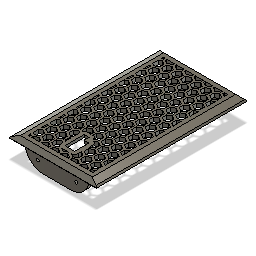
Compact_Robot_MB4 v1 (Autodesk Fusion 360 design; units mm, degrees)
Autodesk Fusion 360 part; units mm, degrees
(part 1 of 2)
sketch "Sketch1" plane through (0, 0, 0) normal (0, 1, 0) x (1, 0, 0)
  line L0 (23.335, 40.235) -> (-23.335, 40.235)
  line L1 (-23.335, 40.235) -> (-23.335, -40.235)
  line L2 (-23.335, -40.235) -> (23.335, -40.235)
  line L3 (23.335, -40.235) -> (23.335, 40.235)
  line L4 (23.335, 40.235) -> (-23.335, -40.235) construction
  line L5 (-23.335, 40.235) -> (23.335, -40.235) construction
  dimension "d1" = 80.47
  dimension "d2" = 46.67
  constraint horizontal L0
  constraint perpendicular L0 L1
  constraint parallel L0 L2
  constraint parallel L1 L3
  constraint coincident L4 origin
  constraint coincident L5 origin
  measures "d1" distance of L0.end L1.end
  measures "d2" distance of L1.end L2.end
extrude "Extrude1" add sketch "Sketch1" along normal blind 2.12
sketch "Sketch2" plane through (0, 0, 0) normal (0, 0, 1) x (1, 0, 0)
  line L0 (-27, 0) -> (28.2654, 0)
  circle A0 centre (-7.215, 0) radius 10
  circle A1 centre (7.215, 0) radius 10
  line L1 (-7.215, -10) -> (7.215, -10)
  line L2 (23.335, 0) -> (23.335, 2.12)
  circle A2 centre (10.2519, -5) radius 0.75
  circle A3 centre (-10.2581, -5) radius 0.75
  dimension "d5" = 20
  dimension "d6" = 20
  dimension "d7" = 14.43
  dimension "d8" = 16.12
  dimension "d12" = 1.5
  dimension "d13" = 1.5
  dimension "d14" = 10
  dimension "d15" = 10
  dimension "d16" = 20.51
  dimension "d17" = 5.85
  constraint horizontal L0
  constraint coincident L0 A0.centre
  constraint coincident L0 A1.centre
  constraint horizontal origin A0.centre
  constraint coincident A1 L1.end
  constraint tangent A1 L1
  constraint tangent A0 L1
  constraint coincident A0 L1.start
  measures "d5" diameter of A0
  measures "d6" diameter of A1
  measures "d7" distance of L1.start L1.end
  measures "d8" distance of A1.centre L2
  measures "d12" diameter of A2
  measures "d13" diameter of A3
  measures "d16" distance of A2.centre A3.centre
  measures "d17" distance of A1.centre A2.centre
extrude "Extrude2" add sketch "Sketch2" along normal blind 1.8 from surface at 36.03 contours L0 A0 A1 | L0 A0 A1 | L0 A0 A1 | A0 A1 L1 picked at (-0.9013, -0.4238) picked at (10.0653, -1.4174) picked at (-10.0674, -1.4174)
extrude "Extrude3" add sketch "Sketch2" along normal blind 1.8 from surface at -37.83 contours L0 A0 A1 | L0 A0 A1 | L0 A0 A1 | A0 A1 L1 picked at (-0.9013, -0.4238) picked at (10.0653, -1.4174) picked at (-10.0674, -1.4174)
sketch "Sketch3" plane through (0, 0, 0) normal (0, 0, 1) x (1, 0, 0)
  line L0 (19.209, 2.12) -> (22.6292, 0.7084)
  line L1 (22.6292, 0.7084) -> (23.335, 0)
  line L2 (-23.335, 2.12) -> (23.335, 2.12)
  line L3 (19.209, 2.12) -> (20.385, 0.1201)
  line L4 (20.385, 0.1201) -> (22.6292, 0.7084)
  line L5 (20.385, 0.1201) -> (20.5053, 0)
  line L6 (-23.335, 0) -> (23.335, 0)
  line L7 (-19.209, 2.12) -> (-22.6292, 0.7084)
  line L8 (-22.6292, 0.7084) -> (-23.335, 0)
  line L9 (-22.6292, 0.7084) -> (-20.385, 0.1201)
  line L10 (-20.385, 0.1201) -> (-19.209, 2.12)
  line L11 (-20.385, 0.1201) -> (-20.5053, 0)
  line L12 (-20.385, 0.1201) -> (20.385, 0.1201)
  line L13 (-23.335, 2.12) -> (-23.335, 0)
  line L14 (-23.335, 2.12) -> (23.335, 2.12)
  line L15 (23.335, 2.12) -> (23.335, 0)
  point P0 (23.335, 0)
  dimension "d21" = 3.7
  dimension "d22" = 1
  dimension "d23" = 2.32
  dimension "d24" = 2.32
  dimension "d25" = 0.17
  dimension "d26" = 3.7
  dimension "d27" = 1
  dimension "d28" = 2.32
  dimension "d29" = 2.32
  dimension "d30" = 0.17
  dimension "d31" = 40.77
  constraint coincident P0 L1.end
  constraint coincident L0.start L2
  constraint coincident L5.end L6
  constraint coincident L2 L7.start
  constraint coincident L6.start L8.end
  constraint coincident L6 L11.end
  constraint horizontal L12
  constraint coincident L2.start L13.start
  constraint coincident L2.end L14.end
  measures "d21" distance of L0.start L0.end
  measures "d22" distance of L0.end P0
  measures "d23" distance of L0.start L3.end
  measures "d24" distance of L0.end L3.end
  measures "d25" distance of L3.end L5.end
  measures "d26" distance of L7.start L7.end
  measures "d27" distance of L7.end L6.start
  measures "d28" distance of L7.end L9.end
  measures "d29" distance of L7.start L9.end
  measures "d30" distance of L9.end L11.end
  measures "d31" horizontal distance of L3.end L9.end
extrude "Extrude4" cut sketch "Sketch3" along normal through all and the other way through all contours L0 L1 L2 L14 L15 | L2 L7 L8 L13 L14
sketch "Sketch4" plane through (0, 0, 0) normal (1, 0, 0) x (0, 0, -1)
  line L0 (-40.235, 0.12) -> (-38.2328, 0.7084)
  line L1 (-40.235, 0.12) -> (-38.2328, 2.12)
  line L2 (-38.2328, 2.12) -> (-38.2328, 0.7084)
  line L3 (40.235, 0.7084) -> (-40.235, 0.7084)
  line L4 (-40.235, 2.12) -> (40.235, 2.12)
  line L5 (-40.235, 0) -> (-40.235, 0.7084)
  line L6 (0, 0) -> (0, 5)
  line L7 (38.2328, 2.12) -> (38.2328, 0.7084)
  line L8 (40.235, 0.12) -> (38.2328, 2.12)
  line L9 (40.235, 0.12) -> (38.2328, 0.7084)
  line L10 (-40.235, 0.12) -> (-40.235, 2.12)
  line L11 (-38.2328, 2.12) -> (-40.235, 2.12)
  line L12 (40.235, 0.12) -> (40.235, 2.12)
  line L13 (38.2328, 2.12) -> (40.235, 2.12)
  dimension "d34" = 2.83
  dimension "d36" = 0.12
  constraint vertical L2
  constraint coincident L0.end L3
  constraint coincident L1.end L4
  constraint coincident L0.start L5
  constraint coincident L0.start L1.start
  constraint coincident L6.start origin
  constraint perpendicular L4 L6
  constraint symmetric L0.start L6 L8.start
  constraint symmetric L0.end L6 L7.end
  constraint symmetric L1.end L6 L7.start
  constraint coincident L4.start L10.end
  constraint coincident L4.end L12.end
  measures "d34" distance of L0.start L1.end
  measures "d36" distance of L0.start L5.start
extrude "Extrude5" cut sketch "Sketch4" along normal through all and the other way through all contours L1 L3 L5 L10 | L1 L3 L4 L10 L11 | L3 L4 L8 L12 L13 | L3 L8 L12
sketch "Sketch5" plane through (0, 2.12, 0) normal (0, 1, 0) x (-1, 0, 0)
  line L0 (-19.209, -38.2328) -> (19.209, -38.2328)
  line L1 (19.209, -38.2328) -> (19.209, 38.2328)
  line L2 (19.209, 38.2328) -> (-19.209, 38.2328)
  line L3 (-19.209, 38.2328) -> (-19.209, -38.2328)
  line L4 (-17.21, -36.03) -> (17.21, -36.03)
  line L5 (17.21, -36.03) -> (17.21, 36.03)
  line L6 (17.21, 36.03) -> (-17.21, 36.03)
  line L7 (-17.21, 36.03) -> (-17.21, -36.03)
  line L8 (-17.21, -36.03) -> (17.21, 36.03) construction
  line L9 (17.21, -36.03) -> (-17.21, 36.03) construction
  line L10 (-0.69, -20.08) -> (3.31, -20.08)
  line L11 (3.31, -20.08) -> (3.31, -31.73)
  line L12 (3.31, -31.73) -> (-3.29, -31.73)
  line L13 (-3.29, -31.73) -> (-3.29, -22.73)
  line L14 (2.61, -20.78) -> (0.01, -20.78)
  line L15 (0.01, -20.78) -> (0.01, -23.43)
  line L16 (2.61, -31.03) -> (2.61, -20.78)
  line L17 (2.61, -31.03) -> (-2.59, -31.03)
  line L18 (-2.59, -31.03) -> (-2.59, -23.43)
  line L19 (-2.59, -23.43) -> (0.01, -23.43)
  line L20 (-3.29, -22.73) -> (-0.69, -22.73)
  line L21 (-0.69, -22.73) -> (-0.69, -20.08)
  line L22 (25, 0) -> (0, 0)
  line L23 (2.61, 31.03) -> (2.61, 20.78)
  line L24 (-2.59, 31.03) -> (-2.59, 23.43)
  line L25 (-0.69, 22.73) -> (-0.69, 20.08)
  line L26 (0.01, 20.78) -> (0.01, 23.43)
  line L27 (3.31, 20.08) -> (3.31, 31.73)
  line L28 (2.61, 20.78) -> (0.01, 20.78)
  line L29 (-3.29, 31.73) -> (-3.29, 22.73)
  line L30 (-2.59, 23.43) -> (0.01, 23.43)
  line L31 (2.61, 31.03) -> (-2.59, 31.03)
  line L32 (-3.29, 22.73) -> (-0.69, 22.73)
  line L33 (3.31, 31.73) -> (-3.29, 31.73)
  line L34 (-0.69, 20.08) -> (3.31, 20.08)
  line L35 (2.61, 33.03) -> (-2.59, 33.03)
  line L36 (-4.59, 31.03) -> (-4.59, 23.43)
  line L37 (-1.99, 21.43) -> (-2.59, 21.43)
  line L38 (-1.99, 21.43) -> (-1.99, 20.78)
  line L39 (4.61, 31.03) -> (4.61, 20.78)
  line L40 (2.61, 18.78) -> (0.01, 18.78)
  arc A0 (4.61, 31.03) -> (2.61, 33.03) centre (2.61, 31.03) ccw
  arc A1 (2.61, 18.78) -> (4.61, 20.78) centre (2.61, 20.78) ccw
  arc A2 (-1.99, 20.78) -> (0.01, 18.78) centre (0.01, 20.78) ccw
  arc A3 (-4.59, 23.43) -> (-2.59, 21.43) centre (-2.59, 23.43) ccw
  arc A4 (-2.59, 33.03) -> (-4.59, 31.03) centre (-2.59, 31.03) ccw
  dimension "d40" = 72.06
  dimension "d41" = 34.42
  dimension "d42" = 0.7
  dimension "d44" = 0.7
  dimension "d46" = 0.7
  dimension "d47" = 0.7
  dimension "d49" = 2.6
  dimension "d51" = 0.7
  dimension "d52" = 7.6
  dimension "d53" = 0.7
  dimension "d54" = 10.25
  dimension "d55" = 5.2
  dimension "d56" = 5
  dimension "d57" = 14.62
  dimension "d63" = 1.3
  dimension "d64" = 1.3
  dimension "d65" = 1.3
  dimension "d66" = 1.3
  dimension "d67" = 1.3
  dimension "d68" = 1.3
  dimension "d69" = 2
  dimension "d70" = 2
  dimension "d71" = 2
  dimension "d72" = 2
  dimension "d73" = 2
  constraint horizontal L4
  constraint perpendicular L4 L5
  constraint parallel L4 L6
  constraint parallel L5 L7
  constraint coincident L8 L22.end
  constraint coincident L9 L22.end
  constraint coincident L22.end origin
  constraint horizontal L10
  constraint vertical L11
  constraint horizontal L12
  constraint vertical L13
  constraint horizontal L20
  constraint horizontal L14
  constraint vertical L15
  constraint vertical L16
  constraint horizontal L17
  constraint vertical L18
  constraint horizontal L19
  constraint perpendicular L3 L22
  constraint symmetric L11.end L22 L27.end
  constraint symmetric L10.start L22 L25.end
  constraint symmetric L10.end L22 L27.start
  constraint symmetric L12.end L22 L29.start
  constraint symmetric L13.end L22 L29.end
  constraint symmetric L14.start L22 L23.end
  constraint symmetric L14.end L22 L26.start
  constraint symmetric L16.start L22 L23.start
  constraint symmetric L17.end L22 L24.start
  constraint symmetric L18.end L22 L24.end
  constraint symmetric L15.end L22 L26.end
  constraint symmetric L20.end L22 L25.start
  constraint horizontal L35
  constraint perpendicular L6 L36
  constraint horizontal L37
  constraint parallel L25 L38
  constraint vertical L39
  constraint perpendicular L39 L40
  constraint tangent L39 A0
  constraint tangent L40 A1
  constraint tangent L38 A2
  constraint tangent L36 A4
  constraint tangent L35 A0
  constraint tangent L35 A4
  constraint tangent L36 A3
  constraint tangent L40 A2
  constraint tangent L37 A3
  constraint tangent L39 A1
  measures "d40" distance of L4.start L6.end
  measures "d41" distance of L5.end L6.end
  measures "d42" distance of L11 L16
  measures "d44" distance of L10 L14
  measures "d46" distance of L19 L20
  measures "d47" distance of L13 L18
  measures "d49" distance of L15 L16
  measures "d51" distance of L15 L21
  measures "d52" distance of L17 L19
  measures "d53" distance of L12 L17
  measures "d54" distance of L14 L17
  measures "d55" distance of L16 L18
  measures "d56" distance of L4 L17
  measures "d57" distance of L7 L18
  measures "d63" distance of L33 L35
  measures "d64" distance of L27 L39
  measures "d65" distance of L29 L36
  measures "d66" distance of L32 L37
  measures "d67" distance of L25 L38
  measures "d68" distance of L34 L40
  measures "d69" radius of A0
  measures "d70" radius of A1
  measures "d71" radius of A2
  measures "d72" radius of A3
  measures "d73" radius of A4
extrude "Extrude6" cut sketch "Sketch5" against normal through all contours L23 L24 L26 L28 L30 L31
extrude "Extrude7" cut sketch "Sketch5" along normal blind 0.7 from surface at -2.12 contours L25 L27 L29 L32 L33 L34
chamfer "Chamfer1" distance 0.7 angle 45 6 edges at (3.29, 0.7, 27.23) (-0.01, 0.7, 31.73) (-3.31, 0.7, 25.905) (1.99, 0.7, 22.73) (0.69, 0.7, 21.405) (-1.31, 0.7, 20.08)
sketch "Sketch6" plane through (0, 2.12, 0) normal (0, 1, 0) x (-1, 0, 0)
  line L0 (0.01, 20.78) -> (0.01, 23.43)
  line L1 (0.01, 23.43) -> (-2.59, 23.43)
  line L2 (-2.59, 23.43) -> (-2.59, 31.03)
  line L3 (-2.59, 31.03) -> (2.61, 31.03)
  line L4 (2.61, 31.03) -> (2.61, 20.78)
  line L5 (2.61, 20.78) -> (0.01, 20.78)
  line L6 (-19.209, -38.2328) -> (19.209, -38.2328)
  line L7 (19.209, -38.2328) -> (19.209, 38.2328)
  line L8 (19.209, 38.2328) -> (-19.209, 38.2328)
  line L9 (-19.209, 38.2328) -> (-19.209, -38.2328)
  line L10 (17.209, 36.0228) -> (17.209, -36.0228)
  line L11 (17.209, -36.0228) -> (-17.209, -36.0228)
  line L12 (-17.209, -36.0228) -> (-17.209, 36.0228)
  line L13 (-17.209, 36.0228) -> (17.209, 36.0228)
  line L14 (16.459, 37.5128) -> (16.459, 35.2028)
  line L15 (16.459, 35.2028) -> (18.4596, 34.0478)
  line L16 (18.4596, 34.0478) -> (20.4601, 35.2028)
  line L17 (20.4601, 35.2028) -> (20.4601, 37.5128)
  line L18 (20.4601, 37.5128) -> (18.4596, 38.6678)
  line L19 (18.4596, 38.6678) -> (16.459, 37.5128)
  line L20 (16.459, 28.4168) -> (16.459, 26.1068)
  line L21 (16.459, 26.1068) -> (18.4596, 24.9518)
  line L22 (18.4596, 24.9518) -> (20.4601, 26.1068)
  line L23 (20.4601, 26.1068) -> (20.4601, 28.4168)
  line L24 (20.4601, 28.4168) -> (18.4596, 29.5718)
  line L25 (18.4596, 29.5718) -> (16.459, 28.4168)
  line L26 (18.4596, 20.4758) -> (16.459, 19.3208)
  line L27 (16.459, 19.3208) -> (16.459, 17.0108)
  line L28 (16.459, 17.0108) -> (18.4596, 15.8558)
  line L29 (18.4596, 15.8558) -> (20.4601, 17.0108)
  line L30 (20.4601, 17.0108) -> (20.4601, 19.3208)
  line L31 (20.4601, 19.3208) -> (18.4596, 20.4758)
  line L32 (18.4596, 11.3798) -> (16.459, 10.2248)
  line L33 (16.459, 10.2248) -> (16.459, 7.9148)
  line L34 (16.459, 7.9148) -> (18.4596, 6.7598)
  line L35 (18.4596, 6.7598) -> (20.4601, 7.9148)
  line L36 (20.4601, 7.9148) -> (20.4601, 10.2248)
  line L37 (20.4601, 10.2248) -> (18.4596, 11.3798)
  line L38 (18.4596, 2.2838) -> (16.459, 1.1288)
  line L39 (16.459, 1.1288) -> (16.459, -1.1812)
  line L40 (16.459, -1.1812) -> (18.4596, -2.3362)
  line L41 (18.4596, -2.3362) -> (20.4601, -1.1812)
  line L42 (20.4601, -1.1812) -> (20.4601, 1.1288)
  line L43 (20.4601, 1.1288) -> (18.4596, 2.2838)
  line L44 (18.4596, -6.8122) -> (16.459, -7.9672)
  line L45 (16.459, -7.9672) -> (16.459, -10.2772)
  line L46 (16.459, -10.2772) -> (18.4596, -11.4322)
  line L47 (18.4596, -11.4322) -> (20.4601, -10.2772)
  line L48 (20.4601, -10.2772) -> (20.4601, -7.9672)
  line L49 (20.4601, -7.9672) -> (18.4596, -6.8122)
  line L50 (18.4596, -15.9082) -> (16.459, -17.0632)
  line L51 (16.459, -17.0632) -> (16.459, -19.3732)
  line L52 (16.459, -19.3732) -> (18.4596, -20.5282)
  line L53 (18.4596, -20.5282) -> (20.4601, -19.3732)
  line L54 (20.4601, -19.3732) -> (20.4601, -17.0632)
  line L55 (20.4601, -17.0632) -> (18.4596, -15.9082)
  line L56 (18.4596, -25.0042) -> (16.459, -26.1592)
  line L57 (16.459, -26.1592) -> (16.459, -28.4692)
  line L58 (16.459, -28.4692) -> (18.4596, -29.6242)
  line L59 (18.4596, -29.6242) -> (20.4601, -28.4692)
  line L60 (20.4601, -28.4692) -> (20.4601, -26.1592)
  line L61 (20.4601, -26.1592) -> (18.4596, -25.0042)
  line L62 (18.4596, -34.1002) -> (16.459, -35.2552)
  line L63 (16.459, -35.2552) -> (16.459, -37.5652)
  line L64 (16.459, -37.5652) -> (18.4596, -38.7202)
  line L65 (18.4596, -38.7202) -> (20.4601, -37.5652)
  line L66 (20.4601, -37.5652) -> (20.4601, -35.2552)
  line L67 (20.4601, -35.2552) -> (18.4596, -34.1002)
  line L68 (13.3396, 29.5718) -> (11.339, 28.4168)
  line L69 (11.339, 28.4168) -> (11.339, 26.1068)
  line L70 (11.339, 26.1068) -> (13.3396, 24.9518)
  line L71 (13.3396, 24.9518) -> (15.3401, 26.1068)
  line L72 (15.3401, 26.1068) -> (15.3401, 28.4168)
  line L73 (15.3401, 28.4168) -> (13.3396, 29.5718)
  line L74 (13.3396, 38.6678) -> (11.339, 37.5128)
  line L75 (11.339, 37.5128) -> (11.339, 35.2028)
  line L76 (11.339, 35.2028) -> (13.3396, 34.0478)
  line L77 (13.3396, 34.0478) -> (15.3401, 35.2028)
  line L78 (15.3401, 35.2028) -> (15.3401, 37.5128)
  line L79 (15.3401, 37.5128) -> (13.3396, 38.6678)
  line L80 (8.2196, 29.5718) -> (6.219, 28.4168)
  line L81 (6.219, 28.4168) -> (6.219, 26.1068)
  line L82 (6.219, 26.1068) -> (8.2196, 24.9518)
  line L83 (8.2196, 24.9518) -> (10.2201, 26.1068)
  line L84 (10.2201, 26.1068) -> (10.2201, 28.4168)
  line L85 (10.2201, 28.4168) -> (8.2196, 29.5718)
  line L86 (8.2196, 38.6678) -> (6.219, 37.5128)
  line L87 (6.219, 37.5128) -> (6.219, 35.2028)
  line L88 (6.219, 35.2028) -> (8.2196, 34.0478)
  line L89 (8.2196, 34.0478) -> (10.2201, 35.2028)
  line L90 (10.2201, 35.2028) -> (10.2201, 37.5128)
  line L91 (10.2201, 37.5128) -> (8.2196, 38.6678)
  line L92 (3.0996, 29.5718) -> (1.099, 28.4168)
  line L93 (1.099, 28.4168) -> (1.099, 26.1068)
  line L94 (1.099, 26.1068) -> (3.0996, 24.9518)
  line L95 (3.0996, 24.9518) -> (5.1001, 26.1068)
  line L96 (5.1001, 26.1068) -> (5.1001, 28.4168)
  line L97 (5.1001, 28.4168) -> (3.0996, 29.5718)
  line L98 (3.0996, 38.6678) -> (1.099, 37.5128)
  line L99 (1.099, 37.5128) -> (1.099, 35.2028)
  line L100 (1.099, 35.2028) -> (3.0996, 34.0478)
  line L101 (3.0996, 34.0478) -> (5.1001, 35.2028)
  line L102 (5.1001, 35.2028) -> (5.1001, 37.5128)
  line L103 (5.1001, 37.5128) -> (3.0996, 38.6678)
  line L104 (-2.0204, 29.5718) -> (-4.021, 28.4168)
  line L105 (-4.021, 28.4168) -> (-4.021, 26.1068)
  line L106 (-4.021, 26.1068) -> (-2.0204, 24.9518)
  line L107 (-2.0204, 24.9518) -> (-0.0199, 26.1068)
  line L108 (-0.0199, 26.1068) -> (-0.0199, 28.4168)
  line L109 (-0.0199, 28.4168) -> (-2.0204, 29.5718)
  line L110 (-2.0204, 38.6678) -> (-4.021, 37.5128)
  line L111 (-4.021, 37.5128) -> (-4.021, 35.2028)
  line L112 (-4.021, 35.2028) -> (-2.0204, 34.0478)
  line L113 (-2.0204, 34.0478) -> (-0.0199, 35.2028)
  line L114 (-0.0199, 35.2028) -> (-0.0199, 37.5128)
  line L115 (-0.0199, 37.5128) -> (-2.0204, 38.6678)
  line L116 (-7.1404, 29.5718) -> (-9.141, 28.4168)
  line L117 (-9.141, 28.4168) -> (-9.141, 26.1068)
  line L118 (-9.141, 26.1068) -> (-7.1404, 24.9518)
  line L119 (-7.1404, 24.9518) -> (-5.1399, 26.1068)
  line L120 (-5.1399, 26.1068) -> (-5.1399, 28.4168)
  line L121 (-5.1399, 28.4168) -> (-7.1404, 29.5718)
  line L122 (-7.1404, 38.6678) -> (-9.141, 37.5128)
  line L123 (-9.141, 37.5128) -> (-9.141, 35.2028)
  line L124 (-9.141, 35.2028) -> (-7.1404, 34.0478)
  line L125 (-7.1404, 34.0478) -> (-5.1399, 35.2028)
  line L126 (-5.1399, 35.2028) -> (-5.1399, 37.5128)
  line L127 (-5.1399, 37.5128) -> (-7.1404, 38.6678)
  line L128 (-12.2604, 29.5718) -> (-14.261, 28.4168)
  line L129 (-14.261, 28.4168) -> (-14.261, 26.1068)
  line L130 (-14.261, 26.1068) -> (-12.2604, 24.9518)
  line L131 (-12.2604, 24.9518) -> (-10.2599, 26.1068)
  line L132 (-10.2599, 26.1068) -> (-10.2599, 28.4168)
  line L133 (-10.2599, 28.4168) -> (-12.2604, 29.5718)
  line L134 (-12.2604, 38.6678) -> (-14.261, 37.5128)
  line L135 (-14.261, 37.5128) -> (-14.261, 35.2028)
  line L136 (-14.261, 35.2028) -> (-12.2604, 34.0478)
  line L137 (-12.2604, 34.0478) -> (-10.2599, 35.2028)
  line L138 (-10.2599, 35.2028) -> (-10.2599, 37.5128)
  line L139 (-10.2599, 37.5128) -> (-12.2604, 38.6678)
  line L140 (-17.3804, 29.5718) -> (-19.381, 28.4168)
  line L141 (-19.381, 28.4168) -> (-19.381, 26.1068)
  line L142 (-19.381, 26.1068) -> (-17.3804, 24.9518)
  line L143 (-17.3804, 24.9518) -> (-15.3799, 26.1068)
  line L144 (-15.3799, 26.1068) -> (-15.3799, 28.4168)
  line L145 (-15.3799, 28.4168) -> (-17.3804, 29.5718)
  line L146 (-17.3804, 38.6678) -> (-19.381, 37.5128)
  line L147 (-19.381, 37.5128) -> (-19.381, 35.2028)
  line L148 (-19.381, 35.2028) -> (-17.3804, 34.0478)
  line L149 (-17.3804, 34.0478) -> (-15.3799, 35.2028)
  line L150 (-15.3799, 35.2028) -> (-15.3799, 37.5128)
  line L151 (-15.3799, 37.5128) -> (-17.3804, 38.6678)
  line L152 (18.4596, 29.5718) -> (16.459, 28.4168)
  line L153 (16.459, 28.4168) -> (16.459, 26.1068)
  line L154 (16.459, 26.1068) -> (18.4596, 24.9518)
  line L155 (18.4596, 24.9518) -> (20.4601, 26.1068)
  line L156 (20.4601, 26.1068) -> (20.4601, 28.4168)
  line L157 (20.4601, 28.4168) -> (18.4596, 29.5718)
  line L158 (13.3396, 20.4758) -> (11.339, 19.3208)
  line L159 (11.339, 19.3208) -> (11.339, 17.0108)
  line L160 (11.339, 17.0108) -> (13.3396, 15.8558)
  line L161 (13.3396, 15.8558) -> (15.3401, 17.0108)
  line L162 (15.3401, 17.0108) -> (15.3401, 19.3208)
  line L163 (15.3401, 19.3208) -> (13.3396, 20.4758)
  line L164 (13.3396, 29.5718) -> (11.339, 28.4168)
  line L165 (11.339, 28.4168) -> (11.339, 26.1068)
  line L166 (11.339, 26.1068) -> (13.3396, 24.9518)
  line L167 (13.3396, 24.9518) -> (15.3401, 26.1068)
  line L168 (15.3401, 26.1068) -> (15.3401, 28.4168)
  line L169 (15.3401, 28.4168) -> (13.3396, 29.5718)
  line L170 (8.2196, 20.4758) -> (6.219, 19.3208)
  line L171 (6.219, 19.3208) -> (6.219, 17.0108)
  line L172 (6.219, 17.0108) -> (8.2196, 15.8558)
  line L173 (8.2196, 15.8558) -> (10.2201, 17.0108)
  line L174 (10.2201, 17.0108) -> (10.2201, 19.3208)
  line L175 (10.2201, 19.3208) -> (8.2196, 20.4758)
  line L176 (8.2196, 29.5718) -> (6.219, 28.4168)
  line L177 (6.219, 28.4168) -> (6.219, 26.1068)
  line L178 (6.219, 26.1068) -> (8.2196, 24.9518)
  line L179 (8.2196, 24.9518) -> (10.2201, 26.1068)
  line L180 (10.2201, 26.1068) -> (10.2201, 28.4168)
  line L181 (10.2201, 28.4168) -> (8.2196, 29.5718)
  line L182 (3.0996, 20.4758) -> (1.099, 19.3208)
  line L183 (1.099, 19.3208) -> (1.099, 17.0108)
  line L184 (1.099, 17.0108) -> (3.0996, 15.8558)
  line L185 (3.0996, 15.8558) -> (5.1001, 17.0108)
  line L186 (5.1001, 17.0108) -> (5.1001, 19.3208)
  line L187 (5.1001, 19.3208) -> (3.0996, 20.4758)
  line L188 (3.0996, 29.5718) -> (1.099, 28.4168)
  line L189 (1.099, 28.4168) -> (1.099, 26.1068)
  line L190 (1.099, 26.1068) -> (3.0996, 24.9518)
  line L191 (3.0996, 24.9518) -> (5.1001, 26.1068)
  line L192 (5.1001, 26.1068) -> (5.1001, 28.4168)
  line L193 (5.1001, 28.4168) -> (3.0996, 29.5718)
  line L194 (-2.0204, 20.4758) -> (-4.021, 19.3208)
  line L195 (-4.021, 19.3208) -> (-4.021, 17.0108)
  line L196 (-4.021, 17.0108) -> (-2.0204, 15.8558)
  line L197 (-2.0204, 15.8558) -> (-0.0199, 17.0108)
  line L198 (-0.0199, 17.0108) -> (-0.0199, 19.3208)
  line L199 (-0.0199, 19.3208) -> (-2.0204, 20.4758)
  line L200 (-2.0204, 29.5718) -> (-4.021, 28.4168)
  line L201 (-4.021, 28.4168) -> (-4.021, 26.1068)
  line L202 (-4.021, 26.1068) -> (-2.0204, 24.9518)
  line L203 (-2.0204, 24.9518) -> (-0.0199, 26.1068)
  line L204 (-0.0199, 26.1068) -> (-0.0199, 28.4168)
  line L205 (-0.0199, 28.4168) -> (-2.0204, 29.5718)
  line L206 (-7.1404, 20.4758) -> (-9.141, 19.3208)
  line L207 (-9.141, 19.3208) -> (-9.141, 17.0108)
  line L208 (-9.141, 17.0108) -> (-7.1404, 15.8558)
  line L209 (-7.1404, 15.8558) -> (-5.1399, 17.0108)
  line L210 (-5.1399, 17.0108) -> (-5.1399, 19.3208)
  line L211 (-5.1399, 19.3208) -> (-7.1404, 20.4758)
  line L212 (-7.1404, 29.5718) -> (-9.141, 28.4168)
  line L213 (-9.141, 28.4168) -> (-9.141, 26.1068)
  line L214 (-9.141, 26.1068) -> (-7.1404, 24.9518)
  line L215 (-7.1404, 24.9518) -> (-5.1399, 26.1068)
  line L216 (-5.1399, 26.1068) -> (-5.1399, 28.4168)
  line L217 (-5.1399, 28.4168) -> (-7.1404, 29.5718)
  line L218 (-12.2604, 20.4758) -> (-14.261, 19.3208)
  line L219 (-14.261, 19.3208) -> (-14.261, 17.0108)
  line L220 (-14.261, 17.0108) -> (-12.2604, 15.8558)
  line L221 (-12.2604, 15.8558) -> (-10.2599, 17.0108)
  line L222 (-10.2599, 17.0108) -> (-10.2599, 19.3208)
  line L223 (-10.2599, 19.3208) -> (-12.2604, 20.4758)
  line L224 (-12.2604, 29.5718) -> (-14.261, 28.4168)
  line L225 (-14.261, 28.4168) -> (-14.261, 26.1068)
  line L226 (-14.261, 26.1068) -> (-12.2604, 24.9518)
  line L227 (-12.2604, 24.9518) -> (-10.2599, 26.1068)
  line L228 (-10.2599, 26.1068) -> (-10.2599, 28.4168)
  line L229 (-10.2599, 28.4168) -> (-12.2604, 29.5718)
  line L230 (-17.3804, 20.4758) -> (-19.381, 19.3208)
  line L231 (-19.381, 19.3208) -> (-19.381, 17.0108)
  line L232 (-19.381, 17.0108) -> (-17.3804, 15.8558)
  line L233 (-17.3804, 15.8558) -> (-15.3799, 17.0108)
  line L234 (-15.3799, 17.0108) -> (-15.3799, 19.3208)
  line L235 (-15.3799, 19.3208) -> (-17.3804, 20.4758)
  line L236 (-17.3804, 29.5718) -> (-19.381, 28.4168)
  line L237 (-19.381, 28.4168) -> (-19.381, 26.1068)
  line L238 (-19.381, 26.1068) -> (-17.3804, 24.9518)
  line L239 (-17.3804, 24.9518) -> (-15.3799, 26.1068)
  line L240 (-15.3799, 26.1068) -> (-15.3799, 28.4168)
  line L241 (-15.3799, 28.4168) -> (-17.3804, 29.5718)
  line L242 (18.4596, 20.4758) -> (16.459, 19.3208)
  line L243 (16.459, 19.3208) -> (16.459, 17.0108)
  line L244 (16.459, 17.0108) -> (18.4596, 15.8558)
  line L245 (18.4596, 15.8558) -> (20.4601, 17.0108)
  line L246 (20.4601, 17.0108) -> (20.4601, 19.3208)
  line L247 (20.4601, 19.3208) -> (18.4596, 20.4758)
  line L248 (13.3396, 11.3798) -> (11.339, 10.2248)
  line L249 (11.339, 10.2248) -> (11.339, 7.9148)
  line L250 (11.339, 7.9148) -> (13.3396, 6.7598)
  line L251 (13.3396, 6.7598) -> (15.3401, 7.9148)
  line L252 (15.3401, 7.9148) -> (15.3401, 10.2248)
  line L253 (15.3401, 10.2248) -> (13.3396, 11.3798)
  line L254 (13.3396, 20.4758) -> (11.339, 19.3208)
  line L255 (11.339, 19.3208) -> (11.339, 17.0108)
  line L256 (11.339, 17.0108) -> (13.3396, 15.8558)
  line L257 (13.3396, 15.8558) -> (15.3401, 17.0108)
  line L258 (15.3401, 17.0108) -> (15.3401, 19.3208)
  line L259 (15.3401, 19.3208) -> (13.3396, 20.4758)
  line L260 (8.2196, 11.3798) -> (6.219, 10.2248)
  line L261 (6.219, 10.2248) -> (6.219, 7.9148)
  line L262 (6.219, 7.9148) -> (8.2196, 6.7598)
  line L263 (8.2196, 6.7598) -> (10.2201, 7.9148)
  line L264 (10.2201, 7.9148) -> (10.2201, 10.2248)
  line L265 (10.2201, 10.2248) -> (8.2196, 11.3798)
  line L266 (8.2196, 20.4758) -> (6.219, 19.3208)
  line L267 (6.219, 19.3208) -> (6.219, 17.0108)
  line L268 (6.219, 17.0108) -> (8.2196, 15.8558)
  line L269 (8.2196, 15.8558) -> (10.2201, 17.0108)
  line L270 (10.2201, 17.0108) -> (10.2201, 19.3208)
  line L271 (10.2201, 19.3208) -> (8.2196, 20.4758)
  line L272 (3.0996, 11.3798) -> (1.099, 10.2248)
  line L273 (1.099, 10.2248) -> (1.099, 7.9148)
  line L274 (1.099, 7.9148) -> (3.0996, 6.7598)
  line L275 (3.0996, 6.7598) -> (5.1001, 7.9148)
  line L276 (5.1001, 7.9148) -> (5.1001, 10.2248)
  line L277 (5.1001, 10.2248) -> (3.0996, 11.3798)
  line L278 (3.0996, 20.4758) -> (1.099, 19.3208)
  line L279 (1.099, 19.3208) -> (1.099, 17.0108)
  line L280 (1.099, 17.0108) -> (3.0996, 15.8558)
  line L281 (3.0996, 15.8558) -> (5.1001, 17.0108)
  line L282 (5.1001, 17.0108) -> (5.1001, 19.3208)
  line L283 (5.1001, 19.3208) -> (3.0996, 20.4758)
  line L284 (-2.0204, 11.3798) -> (-4.021, 10.2248)
  line L285 (-4.021, 10.2248) -> (-4.021, 7.9148)
  line L286 (-4.021, 7.9148) -> (-2.0204, 6.7598)
  line L287 (-2.0204, 6.7598) -> (-0.0199, 7.9148)
  line L288 (-0.0199, 7.9148) -> (-0.0199, 10.2248)
  line L289 (-0.0199, 10.2248) -> (-2.0204, 11.3798)
  line L290 (-2.0204, 20.4758) -> (-4.021, 19.3208)
  line L291 (-4.021, 19.3208) -> (-4.021, 17.0108)
  line L292 (-4.021, 17.0108) -> (-2.0204, 15.8558)
  line L293 (-2.0204, 15.8558) -> (-0.0199, 17.0108)
  line L294 (-0.0199, 17.0108) -> (-0.0199, 19.3208)
  line L295 (-0.0199, 19.3208) -> (-2.0204, 20.4758)
  line L296 (-7.1404, 11.3798) -> (-9.141, 10.2248)
  line L297 (-9.141, 10.2248) -> (-9.141, 7.9148)
  line L298 (-9.141, 7.9148) -> (-7.1404, 6.7598)
  line L299 (-7.1404, 6.7598) -> (-5.1399, 7.9148)
  line L300 (-5.1399, 7.9148) -> (-5.1399, 10.2248)
  line L301 (-5.1399, 10.2248) -> (-7.1404, 11.3798)
  line L302 (-7.1404, 20.4758) -> (-9.141, 19.3208)
  line L303 (-9.141, 19.3208) -> (-9.141, 17.0108)
  line L304 (-9.141, 17.0108) -> (-7.1404, 15.8558)
  line L305 (-7.1404, 15.8558) -> (-5.1399, 17.0108)
  line L306 (-5.1399, 17.0108) -> (-5.1399, 19.3208)
  line L307 (-5.1399, 19.3208) -> (-7.1404, 20.4758)
  line L308 (-12.2604, 11.3798) -> (-14.261, 10.2248)
  line L309 (-14.261, 10.2248) -> (-14.261, 7.9148)
  line L310 (-14.261, 7.9148) -> (-12.2604, 6.7598)
  line L311 (-12.2604, 6.7598) -> (-10.2599, 7.9148)
  line L312 (-10.2599, 7.9148) -> (-10.2599, 10.2248)
  line L313 (-10.2599, 10.2248) -> (-12.2604, 11.3798)
  line L314 (-12.2604, 20.4758) -> (-14.261, 19.3208)
  line L315 (-14.261, 19.3208) -> (-14.261, 17.0108)
  line L316 (-14.261, 17.0108) -> (-12.2604, 15.8558)
  line L317 (-12.2604, 15.8558) -> (-10.2599, 17.0108)
  line L318 (-10.2599, 17.0108) -> (-10.2599, 19.3208)
  line L319 (-10.2599, 19.3208) -> (-12.2604, 20.4758)
  line L320 (-17.3804, 11.3798) -> (-19.381, 10.2248)
  line L321 (-19.381, 10.2248) -> (-19.381, 7.9148)
  line L322 (-19.381, 7.9148) -> (-17.3804, 6.7598)
  line L323 (-17.3804, 6.7598) -> (-15.3799, 7.9148)
  line L324 (-15.3799, 7.9148) -> (-15.3799, 10.2248)
  line L325 (-15.3799, 10.2248) -> (-17.3804, 11.3798)
  line L326 (-17.3804, 20.4758) -> (-19.381, 19.3208)
  line L327 (-19.381, 19.3208) -> (-19.381, 17.0108)
  line L328 (-19.381, 17.0108) -> (-17.3804, 15.8558)
  line L329 (-17.3804, 15.8558) -> (-15.3799, 17.0108)
  line L330 (-15.3799, 17.0108) -> (-15.3799, 19.3208)
  line L331 (-15.3799, 19.3208) -> (-17.3804, 20.4758)
  line L332 (18.4596, 11.3798) -> (16.459, 10.2248)
  line L333 (16.459, 10.2248) -> (16.459, 7.9148)
  line L334 (16.459, 7.9148) -> (18.4596, 6.7598)
  line L335 (18.4596, 6.7598) -> (20.4601, 7.9148)
  line L336 (20.4601, 7.9148) -> (20.4601, 10.2248)
  line L337 (20.4601, 10.2248) -> (18.4596, 11.3798)
  line L338 (13.3396, 2.2838) -> (11.339, 1.1288)
  line L339 (11.339, 1.1288) -> (11.339, -1.1812)
  line L340 (11.339, -1.1812) -> (13.3396, -2.3362)
  line L341 (13.3396, -2.3362) -> (15.3401, -1.1812)
  line L342 (15.3401, -1.1812) -> (15.3401, 1.1288)
  line L343 (15.3401, 1.1288) -> (13.3396, 2.2838)
  line L344 (13.3396, 11.3798) -> (11.339, 10.2248)
  line L345 (11.339, 10.2248) -> (11.339, 7.9148)
  line L346 (11.339, 7.9148) -> (13.3396, 6.7598)
  line L347 (13.3396, 6.7598) -> (15.3401, 7.9148)
  line L348 (15.3401, 7.9148) -> (15.3401, 10.2248)
  line L349 (15.3401, 10.2248) -> (13.3396, 11.3798)
  line L350 (8.2196, 2.2838) -> (6.219, 1.1288)
  line L351 (6.219, 1.1288) -> (6.219, -1.1812)
  line L352 (6.219, -1.1812) -> (8.2196, -2.3362)
  line L353 (8.2196, -2.3362) -> (10.2201, -1.1812)
  line L354 (10.2201, -1.1812) -> (10.2201, 1.1288)
  line L355 (10.2201, 1.1288) -> (8.2196, 2.2838)
  line L356 (8.2196, 11.3798) -> (6.219, 10.2248)
  line L357 (6.219, 10.2248) -> (6.219, 7.9148)
  line L358 (6.219, 7.9148) -> (8.2196, 6.7598)
  line L359 (8.2196, 6.7598) -> (10.2201, 7.9148)
  line L360 (10.2201, 7.9148) -> (10.2201, 10.2248)
  line L361 (10.2201, 10.2248) -> (8.2196, 11.3798)
  line L362 (3.0996, 2.2838) -> (1.099, 1.1288)
  line L363 (1.099, 1.1288) -> (1.099, -1.1812)
  line L364 (1.099, -1.1812) -> (3.0996, -2.3362)
  line L365 (3.0996, -2.3362) -> (5.1001, -1.1812)
  line L366 (5.1001, -1.1812) -> (5.1001, 1.1288)
  line L367 (5.1001, 1.1288) -> (3.0996, 2.2838)
  line L368 (3.0996, 11.3798) -> (1.099, 10.2248)
  line L369 (1.099, 10.2248) -> (1.099, 7.9148)
  line L370 (1.099, 7.9148) -> (3.0996, 6.7598)
  line L371 (3.0996, 6.7598) -> (5.1001, 7.9148)
  line L372 (5.1001, 7.9148) -> (5.1001, 10.2248)
  line L373 (5.1001, 10.2248) -> (3.0996, 11.3798)
  line L374 (-2.0204, 2.2838) -> (-4.021, 1.1288)
  line L375 (-4.021, 1.1288) -> (-4.021, -1.1812)
  line L376 (-4.021, -1.1812) -> (-2.0204, -2.3362)
  line L377 (-2.0204, -2.3362) -> (-0.0199, -1.1812)
  line L378 (-0.0199, -1.1812) -> (-0.0199, 1.1288)
  line L379 (-0.0199, 1.1288) -> (-2.0204, 2.2838)
  line L380 (-2.0204, 11.3798) -> (-4.021, 10.2248)
  line L381 (-4.021, 10.2248) -> (-4.021, 7.9148)
  line L382 (-4.021, 7.9148) -> (-2.0204, 6.7598)
  line L383 (-2.0204, 6.7598) -> (-0.0199, 7.9148)
  line L384 (-0.0199, 7.9148) -> (-0.0199, 10.2248)
  line L385 (-0.0199, 10.2248) -> (-2.0204, 11.3798)
  line L386 (-7.1404, 2.2838) -> (-9.141, 1.1288)
  line L387 (-9.141, 1.1288) -> (-9.141, -1.1812)
  line L388 (-9.141, -1.1812) -> (-7.1404, -2.3362)
  line L389 (-7.1404, -2.3362) -> (-5.1399, -1.1812)
  line L390 (-5.1399, -1.1812) -> (-5.1399, 1.1288)
  line L391 (-5.1399, 1.1288) -> (-7.1404, 2.2838)
  line L392 (-7.1404, 11.3798) -> (-9.141, 10.2248)
  line L393 (-9.141, 10.2248) -> (-9.141, 7.9148)
  line L394 (-9.141, 7.9148) -> (-7.1404, 6.7598)
  line L395 (-7.1404, 6.7598) -> (-5.1399, 7.9148)
  line L396 (-5.1399, 7.9148) -> (-5.1399, 10.2248)
  line L397 (-5.1399, 10.2248) -> (-7.1404, 11.3798)
  line L398 (-12.2604, 2.2838) -> (-14.261, 1.1288)
  line L399 (-14.261, 1.1288) -> (-14.261, -1.1812)
  line L400 (-14.261, -1.1812) -> (-12.2604, -2.3362)
  line L401 (-12.2604, -2.3362) -> (-10.2599, -1.1812)
  line L402 (-10.2599, -1.1812) -> (-10.2599, 1.1288)
  line L403 (-10.2599, 1.1288) -> (-12.2604, 2.2838)
  line L404 (-12.2604, 11.3798) -> (-14.261, 10.2248)
  line L405 (-14.261, 10.2248) -> (-14.261, 7.9148)
  line L406 (-14.261, 7.9148) -> (-12.2604, 6.7598)
  line L407 (-12.2604, 6.7598) -> (-10.2599, 7.9148)
  line L408 (-10.2599, 7.9148) -> (-10.2599, 10.2248)
  line L409 (-10.2599, 10.2248) -> (-12.2604, 11.3798)
  line L410 (-17.3804, 2.2838) -> (-19.381, 1.1288)
  line L411 (-19.381, 1.1288) -> (-19.381, -1.1812)
  line L412 (-19.381, -1.1812) -> (-17.3804, -2.3362)
  line L413 (-17.3804, -2.3362) -> (-15.3799, -1.1812)
  line L414 (-15.3799, -1.1812) -> (-15.3799, 1.1288)
  line L415 (-15.3799, 1.1288) -> (-17.3804, 2.2838)
  line L416 (-17.3804, 11.3798) -> (-19.381, 10.2248)
  line L417 (-19.381, 10.2248) -> (-19.381, 7.9148)
  line L418 (-19.381, 7.9148) -> (-17.3804, 6.7598)
  line L419 (-17.3804, 6.7598) -> (-15.3799, 7.9148)
  line L420 (-15.3799, 7.9148) -> (-15.3799, 10.2248)
  line L421 (-15.3799, 10.2248) -> (-17.3804, 11.3798)
  line L422 (18.4596, 2.2838) -> (16.459, 1.1288)
  line L423 (16.459, 1.1288) -> (16.459, -1.1812)
  line L424 (16.459, -1.1812) -> (18.4596, -2.3362)
  line L425 (18.4596, -2.3362) -> (20.4601, -1.1812)
  line L426 (20.4601, -1.1812) -> (20.4601, 1.1288)
  line L427 (20.4601, 1.1288) -> (18.4596, 2.2838)
  line L428 (13.3396, -6.8122) -> (11.339, -7.9672)
  line L429 (11.339, -7.9672) -> (11.339, -10.2772)
  line L430 (11.339, -10.2772) -> (13.3396, -11.4322)
  line L431 (13.3396, -11.4322) -> (15.3401, -10.2772)
  line L432 (15.3401, -10.2772) -> (15.3401, -7.9672)
  line L433 (15.3401, -7.9672) -> (13.3396, -6.8122)
  line L434 (13.3396, 2.2838) -> (11.339, 1.1288)
  line L435 (11.339, 1.1288) -> (11.339, -1.1812)
  line L436 (11.339, -1.1812) -> (13.3396, -2.3362)
  line L437 (13.3396, -2.3362) -> (15.3401, -1.1812)
  line L438 (15.3401, -1.1812) -> (15.3401, 1.1288)
  line L439 (15.3401, 1.1288) -> (13.3396, 2.2838)
  line L440 (8.2196, -6.8122) -> (6.219, -7.9672)
  line L441 (6.219, -7.9672) -> (6.219, -10.2772)
  line L442 (6.219, -10.2772) -> (8.2196, -11.4322)
  line L443 (8.2196, -11.4322) -> (10.2201, -10.2772)
  line L444 (10.2201, -10.2772) -> (10.2201, -7.9672)
  line L445 (10.2201, -7.9672) -> (8.2196, -6.8122)
  line L446 (8.2196, 2.2838) -> (6.219, 1.1288)
  line L447 (6.219, 1.1288) -> (6.219, -1.1812)
  line L448 (6.219, -1.1812) -> (8.2196, -2.3362)
  line L449 (8.2196, -2.3362) -> (10.2201, -1.1812)
  line L450 (10.2201, -1.1812) -> (10.2201, 1.1288)
  line L451 (10.2201, 1.1288) -> (8.2196, 2.2838)
  line L452 (3.0996, -6.8122) -> (1.099, -7.9672)
  line L453 (1.099, -7.9672) -> (1.099, -10.2772)
  line L454 (1.099, -10.2772) -> (3.0996, -11.4322)
  line L455 (3.0996, -11.4322) -> (5.1001, -10.2772)
  line L456 (5.1001, -10.2772) -> (5.1001, -7.9672)
  line L457 (5.1001, -7.9672) -> (3.0996, -6.8122)
  line L458 (3.0996, 2.2838) -> (1.099, 1.1288)
  line L459 (1.099, 1.1288) -> (1.099, -1.1812)
  line L460 (1.099, -1.1812) -> (3.0996, -2.3362)
  line L461 (3.0996, -2.3362) -> (5.1001, -1.1812)
  line L462 (5.1001, -1.1812) -> (5.1001, 1.1288)
  line L463 (5.1001, 1.1288) -> (3.0996, 2.2838)
  line L464 (-2.0204, -6.8122) -> (-4.021, -7.9672)
  line L465 (-4.021, -7.9672) -> (-4.021, -10.2772)
  line L466 (-4.021, -10.2772) -> (-2.0204, -11.4322)
  line L467 (-2.0204, -11.4322) -> (-0.0199, -10.2772)
  line L468 (-0.0199, -10.2772) -> (-0.0199, -7.9672)
  line L469 (-0.0199, -7.9672) -> (-2.0204, -6.8122)
  line L470 (-2.0204, 2.2838) -> (-4.021, 1.1288)
  line L471 (-4.021, 1.1288) -> (-4.021, -1.1812)
  line L472 (-4.021, -1.1812) -> (-2.0204, -2.3362)
  line L473 (-2.0204, -2.3362) -> (-0.0199, -1.1812)
  line L474 (-0.0199, -1.1812) -> (-0.0199, 1.1288)
  line L475 (-0.0199, 1.1288) -> (-2.0204, 2.2838)
  line L476 (-7.1404, -6.8122) -> (-9.141, -7.9672)
  line L477 (-9.141, -7.9672) -> (-9.141, -10.2772)
  line L478 (-9.141, -10.2772) -> (-7.1404, -11.4322)
  line L479 (-7.1404, -11.4322) -> (-5.1399, -10.2772)
  line L480 (-5.1399, -10.2772) -> (-5.1399, -7.9672)
  line L481 (-5.1399, -7.9672) -> (-7.1404, -6.8122)
  line L482 (-7.1404, 2.2838) -> (-9.141, 1.1288)
  line L483 (-9.141, 1.1288) -> (-9.141, -1.1812)
  line L484 (-9.141, -1.1812) -> (-7.1404, -2.3362)
  line L485 (-7.1404, -2.3362) -> (-5.1399, -1.1812)
  line L486 (-5.1399, -1.1812) -> (-5.1399, 1.1288)
  line L487 (-5.1399, 1.1288) -> (-7.1404, 2.2838)
  line L488 (-12.2604, -6.8122) -> (-14.261, -7.9672)
  line L489 (-14.261, -7.9672) -> (-14.261, -10.2772)
  line L490 (-14.261, -10.2772) -> (-12.2604, -11.4322)
  line L491 (-12.2604, -11.4322) -> (-10.2599, -10.2772)
  line L492 (-10.2599, -10.2772) -> (-10.2599, -7.9672)
  line L493 (-10.2599, -7.9672) -> (-12.2604, -6.8122)
  line L494 (-12.2604, 2.2838) -> (-14.261, 1.1288)
  line L495 (-14.261, 1.1288) -> (-14.261, -1.1812)
  line L496 (-14.261, -1.1812) -> (-12.2604, -2.3362)
  line L497 (-12.2604, -2.3362) -> (-10.2599, -1.1812)
  line L498 (-10.2599, -1.1812) -> (-10.2599, 1.1288)
  line L499 (-10.2599, 1.1288) -> (-12.2604, 2.2838)
  line L500 (-17.3804, -6.8122) -> (-19.381, -7.9672)
  line L501 (-19.381, -7.9672) -> (-19.381, -10.2772)
  line L502 (-19.381, -10.2772) -> (-17.3804, -11.4322)
  line L503 (-17.3804, -11.4322) -> (-15.3799, -10.2772)
  line L504 (-15.3799, -10.2772) -> (-15.3799, -7.9672)
  line L505 (-15.3799, -7.9672) -> (-17.3804, -6.8122)
  line L506 (-17.3804, 2.2838) -> (-19.381, 1.1288)
  line L507 (-19.381, 1.1288) -> (-19.381, -1.1812)
  line L508 (-19.381, -1.1812) -> (-17.3804, -2.3362)
  line L509 (-17.3804, -2.3362) -> (-15.3799, -1.1812)
  line L510 (-15.3799, -1.1812) -> (-15.3799, 1.1288)
  line L511 (-15.3799, 1.1288) -> (-17.3804, 2.2838)
  line L512 (18.4596, -6.8122) -> (16.459, -7.9672)
  line L513 (16.459, -7.9672) -> (16.459, -10.2772)
  line L514 (16.459, -10.2772) -> (18.4596, -11.4322)
  line L515 (18.4596, -11.4322) -> (20.4601, -10.2772)
  line L516 (20.4601, -10.2772) -> (20.4601, -7.9672)
  line L517 (20.4601, -7.9672) -> (18.4596, -6.8122)
  line L518 (13.3396, -15.9082) -> (11.339, -17.0632)
  line L519 (11.339, -17.0632) -> (11.339, -19.3732)
  line L520 (11.339, -19.3732) -> (13.3396, -20.5282)
  line L521 (13.3396, -20.5282) -> (15.3401, -19.3732)
  line L522 (15.3401, -19.3732) -> (15.3401, -17.0632)
  line L523 (15.3401, -17.0632) -> (13.3396, -15.9082)
  line L524 (13.3396, -6.8122) -> (11.339, -7.9672)
  line L525 (11.339, -7.9672) -> (11.339, -10.2772)
  line L526 (11.339, -10.2772) -> (13.3396, -11.4322)
  line L527 (13.3396, -11.4322) -> (15.3401, -10.2772)
  line L528 (15.3401, -10.2772) -> (15.3401, -7.9672)
  line L529 (15.3401, -7.9672) -> (13.3396, -6.8122)
  line L530 (8.2196, -15.9082) -> (6.219, -17.0632)
  line L531 (6.219, -17.0632) -> (6.219, -19.3732)
  line L532 (6.219, -19.3732) -> (8.2196, -20.5282)
  line L533 (8.2196, -20.5282) -> (10.2201, -19.3732)
  line L534 (10.2201, -19.3732) -> (10.2201, -17.0632)
  line L535 (10.2201, -17.0632) -> (8.2196, -15.9082)
  line L536 (8.2196, -6.8122) -> (6.219, -7.9672)
  line L537 (6.219, -7.9672) -> (6.219, -10.2772)
  line L538 (6.219, -10.2772) -> (8.2196, -11.4322)
  line L539 (8.2196, -11.4322) -> (10.2201, -10.2772)
  line L540 (10.2201, -10.2772) -> (10.2201, -7.9672)
  line L541 (10.2201, -7.9672) -> (8.2196, -6.8122)
  line L542 (3.0996, -15.9082) -> (1.099, -17.0632)
  line L543 (1.099, -17.0632) -> (1.099, -19.3732)
  line L544 (1.099, -19.3732) -> (3.0996, -20.5282)
  line L545 (3.0996, -20.5282) -> (5.1001, -19.3732)
  line L546 (5.1001, -19.3732) -> (5.1001, -17.0632)
  line L547 (5.1001, -17.0632) -> (3.0996, -15.9082)
  line L548 (3.0996, -6.8122) -> (1.099, -7.9672)
  line L549 (1.099, -7.9672) -> (1.099, -10.2772)
  line L550 (1.099, -10.2772) -> (3.0996, -11.4322)
  line L551 (3.0996, -11.4322) -> (5.1001, -10.2772)
  line L552 (5.1001, -10.2772) -> (5.1001, -7.9672)
  line L553 (5.1001, -7.9672) -> (3.0996, -6.8122)
  line L554 (-2.0204, -15.9082) -> (-4.021, -17.0632)
  line L555 (-4.021, -17.0632) -> (-4.021, -19.3732)
  line L556 (-4.021, -19.3732) -> (-2.0204, -20.5282)
  line L557 (-2.0204, -20.5282) -> (-0.0199, -19.3732)
  line L558 (-0.0199, -19.3732) -> (-0.0199, -17.0632)
  line L559 (-0.0199, -17.0632) -> (-2.0204, -15.9082)
  line L560 (-2.0204, -6.8122) -> (-4.021, -7.9672)
  line L561 (-4.021, -7.9672) -> (-4.021, -10.2772)
  line L562 (-4.021, -10.2772) -> (-2.0204, -11.4322)
  line L563 (-2.0204, -11.4322) -> (-0.0199, -10.2772)
  line L564 (-0.0199, -10.2772) -> (-0.0199, -7.9672)
  line L565 (-0.0199, -7.9672) -> (-2.0204, -6.8122)
  line L566 (-7.1404, -15.9082) -> (-9.141, -17.0632)
  line L567 (-9.141, -17.0632) -> (-9.141, -19.3732)
  line L568 (-9.141, -19.3732) -> (-7.1404, -20.5282)
  line L569 (-7.1404, -20.5282) -> (-5.1399, -19.3732)
  line L570 (-5.1399, -19.3732) -> (-5.1399, -17.0632)
  line L571 (-5.1399, -17.0632) -> (-7.1404, -15.9082)
  line L572 (-7.1404, -6.8122) -> (-9.141, -7.9672)
  line L573 (-9.141, -7.9672) -> (-9.141, -10.2772)
  line L574 (-9.141, -10.2772) -> (-7.1404, -11.4322)
  line L575 (-7.1404, -11.4322) -> (-5.1399, -10.2772)
  line L576 (-5.1399, -10.2772) -> (-5.1399, -7.9672)
  line L577 (-5.1399, -7.9672) -> (-7.1404, -6.8122)
  line L578 (-12.2604, -15.9082) -> (-14.261, -17.0632)
  line L579 (-14.261, -17.0632) -> (-14.261, -19.3732)
  line L580 (-14.261, -19.3732) -> (-12.2604, -20.5282)
  line L581 (-12.2604, -20.5282) -> (-10.2599, -19.3732)
  line L582 (-10.2599, -19.3732) -> (-10.2599, -17.0632)
  line L583 (-10.2599, -17.0632) -> (-12.2604, -15.9082)
  line L584 (-12.2604, -6.8122) -> (-14.261, -7.9672)
  line L585 (-14.261, -7.9672) -> (-14.261, -10.2772)
  line L586 (-14.261, -10.2772) -> (-12.2604, -11.4322)
  line L587 (-12.2604, -11.4322) -> (-10.2599, -10.2772)
  line L588 (-10.2599, -10.2772) -> (-10.2599, -7.9672)
  line L589 (-10.2599, -7.9672) -> (-12.2604, -6.8122)
  line L590 (-17.3804, -15.9082) -> (-19.381, -17.0632)
  line L591 (-19.381, -17.0632) -> (-19.381, -19.3732)
  line L592 (-19.381, -19.3732) -> (-17.3804, -20.5282)
  line L593 (-17.3804, -20.5282) -> (-15.3799, -19.3732)
  line L594 (-15.3799, -19.3732) -> (-15.3799, -17.0632)
  line L595 (-15.3799, -17.0632) -> (-17.3804, -15.9082)
  line L596 (-17.3804, -6.8122) -> (-19.381, -7.9672)
  line L597 (-19.381, -7.9672) -> (-19.381, -10.2772)
  line L598 (-19.381, -10.2772) -> (-17.3804, -11.4322)
  line L599 (-17.3804, -11.4322) -> (-15.3799, -10.2772)
  line L600 (-15.3799, -10.2772) -> (-15.3799, -7.9672)
  line L601 (-15.3799, -7.9672) -> (-17.3804, -6.8122)
  line L602 (18.4596, -15.9082) -> (16.459, -17.0632)
  line L603 (16.459, -17.0632) -> (16.459, -19.3732)
  line L604 (16.459, -19.3732) -> (18.4596, -20.5282)
  line L605 (18.4596, -20.5282) -> (20.4601, -19.3732)
  line L606 (20.4601, -19.3732) -> (20.4601, -17.0632)
  line L607 (20.4601, -17.0632) -> (18.4596, -15.9082)
  line L608 (13.3396, -25.0042) -> (11.339, -26.1592)
  line L609 (11.339, -26.1592) -> (11.339, -28.4692)
  line L610 (11.339, -28.4692) -> (13.3396, -29.6242)
  line L611 (13.3396, -29.6242) -> (15.3401, -28.4692)
  line L612 (15.3401, -28.4692) -> (15.3401, -26.1592)
  line L613 (15.3401, -26.1592) -> (13.3396, -25.0042)
  line L614 (13.3396, -15.9082) -> (11.339, -17.0632)
  line L615 (11.339, -17.0632) -> (11.339, -19.3732)
  line L616 (11.339, -19.3732) -> (13.3396, -20.5282)
  line L617 (13.3396, -20.5282) -> (15.3401, -19.3732)
  line L618 (15.3401, -19.3732) -> (15.3401, -17.0632)
  line L619 (15.3401, -17.0632) -> (13.3396, -15.9082)
  line L620 (8.2196, -25.0042) -> (6.219, -26.1592)
  line L621 (6.219, -26.1592) -> (6.219, -28.4692)
  line L622 (6.219, -28.4692) -> (8.2196, -29.6242)
  line L623 (8.2196, -29.6242) -> (10.2201, -28.4692)
  line L624 (10.2201, -28.4692) -> (10.2201, -26.1592)
  line L625 (10.2201, -26.1592) -> (8.2196, -25.0042)
  line L626 (8.2196, -15.9082) -> (6.219, -17.0632)
  line L627 (6.219, -17.0632) -> (6.219, -19.3732)
  line L628 (6.219, -19.3732) -> (8.2196, -20.5282)
  line L629 (8.2196, -20.5282) -> (10.2201, -19.3732)
  line L630 (10.2201, -19.3732) -> (10.2201, -17.0632)
  line L631 (10.2201, -17.0632) -> (8.2196, -15.9082)
  line L632 (3.0996, -25.0042) -> (1.099, -26.1592)
  line L633 (1.099, -26.1592) -> (1.099, -28.4692)
  line L634 (1.099, -28.4692) -> (3.0996, -29.6242)
  line L635 (3.0996, -29.6242) -> (5.1001, -28.4692)
  line L636 (5.1001, -28.4692) -> (5.1001, -26.1592)
  line L637 (5.1001, -26.1592) -> (3.0996, -25.0042)
  line L638 (3.0996, -15.9082) -> (1.099, -17.0632)
  line L639 (1.099, -17.0632) -> (1.099, -19.3732)
  line L640 (1.099, -19.3732) -> (3.0996, -20.5282)
  line L641 (3.0996, -20.5282) -> (5.1001, -19.3732)
  line L642 (5.1001, -19.3732) -> (5.1001, -17.0632)
  line L643 (5.1001, -17.0632) -> (3.0996, -15.9082)
  line L644 (-2.0204, -25.0042) -> (-4.021, -26.1592)
  line L645 (-4.021, -26.1592) -> (-4.021, -28.4692)
  line L646 (-4.021, -28.4692) -> (-2.0204, -29.6242)
  line L647 (-2.0204, -29.6242) -> (-0.0199, -28.4692)
  line L648 (-0.0199, -28.4692) -> (-0.0199, -26.1592)
  line L649 (-0.0199, -26.1592) -> (-2.0204, -25.0042)
  line L650 (-2.0204, -15.9082) -> (-4.021, -17.0632)
  line L651 (-4.021, -17.0632) -> (-4.021, -19.3732)
  line L652 (-4.021, -19.3732) -> (-2.0204, -20.5282)
  line L653 (-2.0204, -20.5282) -> (-0.0199, -19.3732)
  line L654 (-0.0199, -19.3732) -> (-0.0199, -17.0632)
  line L655 (-0.0199, -17.0632) -> (-2.0204, -15.9082)
  line L656 (-7.1404, -25.0042) -> (-9.141, -26.1592)
  line L657 (-9.141, -26.1592) -> (-9.141, -28.4692)
  line L658 (-9.141, -28.4692) -> (-7.1404, -29.6242)
  line L659 (-7.1404, -29.6242) -> (-5.1399, -28.4692)
  line L660 (-5.1399, -28.4692) -> (-5.1399, -26.1592)
  line L661 (-5.1399, -26.1592) -> (-7.1404, -25.0042)
  line L662 (-7.1404, -15.9082) -> (-9.141, -17.0632)
  line L663 (-9.141, -17.0632) -> (-9.141, -19.3732)
  line L664 (-9.141, -19.3732) -> (-7.1404, -20.5282)
  line L665 (-7.1404, -20.5282) -> (-5.1399, -19.3732)
  line L666 (-5.1399, -19.3732) -> (-5.1399, -17.0632)
  line L667 (-5.1399, -17.0632) -> (-7.1404, -15.9082)
  line L668 (-12.2604, -25.0042) -> (-14.261, -26.1592)
  line L669 (-14.261, -26.1592) -> (-14.261, -28.4692)
  line L670 (-14.261, -28.4692) -> (-12.2604, -29.6242)
  line L671 (-12.2604, -29.6242) -> (-10.2599, -28.4692)
  line L672 (-10.2599, -28.4692) -> (-10.2599, -26.1592)
  line L673 (-10.2599, -26.1592) -> (-12.2604, -25.0042)
  line L674 (-12.2604, -15.9082) -> (-14.261, -17.0632)
  line L675 (-14.261, -17.0632) -> (-14.261, -19.3732)
  line L676 (-14.261, -19.3732) -> (-12.2604, -20.5282)
  line L677 (-12.2604, -20.5282) -> (-10.2599, -19.3732)
  line L678 (-10.2599, -19.3732) -> (-10.2599, -17.0632)
  line L679 (-10.2599, -17.0632) -> (-12.2604, -15.9082)
  line L680 (-17.3804, -25.0042) -> (-19.381, -26.1592)
  line L681 (-19.381, -26.1592) -> (-19.381, -28.4692)
  line L682 (-19.381, -28.4692) -> (-17.3804, -29.6242)
  line L683 (-17.3804, -29.6242) -> (-15.3799, -28.4692)
  line L684 (-15.3799, -28.4692) -> (-15.3799, -26.1592)
  line L685 (-15.3799, -26.1592) -> (-17.3804, -25.0042)
  line L686 (-17.3804, -15.9082) -> (-19.381, -17.0632)
  line L687 (-19.381, -17.0632) -> (-19.381, -19.3732)
  line L688 (-19.381, -19.3732) -> (-17.3804, -20.5282)
  line L689 (-17.3804, -20.5282) -> (-15.3799, -19.3732)
  line L690 (-15.3799, -19.3732) -> (-15.3799, -17.0632)
  line L691 (-15.3799, -17.0632) -> (-17.3804, -15.9082)
  line L692 (18.4596, -25.0042) -> (16.459, -26.1592)
  line L693 (16.459, -26.1592) -> (16.459, -28.4692)
  line L694 (16.459, -28.4692) -> (18.4596, -29.6242)
  line L695 (18.4596, -29.6242) -> (20.4601, -28.4692)
  line L696 (20.4601, -28.4692) -> (20.4601, -26.1592)
  line L697 (20.4601, -26.1592) -> (18.4596, -25.0042)
  line L698 (13.3396, -34.1002) -> (11.339, -35.2552)
  line L699 (11.339, -35.2552) -> (11.339, -37.5652)
  line L700 (11.339, -37.5652) -> (13.3396, -38.7202)
  line L701 (13.3396, -38.7202) -> (15.3401, -37.5652)
  line L702 (15.3401, -37.5652) -> (15.3401, -35.2552)
  line L703 (15.3401, -35.2552) -> (13.3396, -34.1002)
  line L704 (13.3396, -25.0042) -> (11.339, -26.1592)
  line L705 (11.339, -26.1592) -> (11.339, -28.4692)
  line L706 (11.339, -28.4692) -> (13.3396, -29.6242)
  line L707 (13.3396, -29.6242) -> (15.3401, -28.4692)
  line L708 (15.3401, -28.4692) -> (15.3401, -26.1592)
  line L709 (15.3401, -26.1592) -> (13.3396, -25.0042)
  line L710 (8.2196, -34.1002) -> (6.219, -35.2552)
  line L711 (6.219, -35.2552) -> (6.219, -37.5652)
  line L712 (6.219, -37.5652) -> (8.2196, -38.7202)
  line L713 (8.2196, -38.7202) -> (10.2201, -37.5652)
  line L714 (10.2201, -37.5652) -> (10.2201, -35.2552)
  line L715 (10.2201, -35.2552) -> (8.2196, -34.1002)
  line L716 (8.2196, -25.0042) -> (6.219, -26.1592)
  line L717 (6.219, -26.1592) -> (6.219, -28.4692)
  line L718 (6.219, -28.4692) -> (8.2196, -29.6242)
  line L719 (8.2196, -29.6242) -> (10.2201, -28.4692)
  line L720 (10.2201, -28.4692) -> (10.2201, -26.1592)
  line L721 (10.2201, -26.1592) -> (8.2196, -25.0042)
  line L722 (3.0996, -34.1002) -> (1.099, -35.2552)
  line L723 (1.099, -35.2552) -> (1.099, -37.5652)
  line L724 (1.099, -37.5652) -> (3.0996, -38.7202)
  line L725 (3.0996, -38.7202) -> (5.1001, -37.5652)